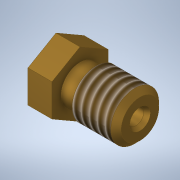
# Autodesk Inventor part: MINI-nozzle-0.4
Saved by Autodesk Inventor 2021 (Build 250183000, 183)
## iProperties
Company: Prusa Development a.s.
Created: 2019-02-18
Material: Všeobecné
Document SubType Name: Modeling
Density: 1 g/cm^3
Appearance: Mosaz – satén
Project: ORIGINAL PRUSA MINI
Authority: Ing. Robert Turinský
Author: Ing. Robert Turinský
Title: MINI-nozzle-0.4
Revision Number: R4
Autodesk Inventor part; units mm, degrees
ref_plane "YZ Plane" through (0, 0, 0) normal (1, 0, 0) x (0, 1, 0)
ref_plane "XZ Plane" through (0, 0, 0) normal (0, 1, 0) x (-1, 0, 0)
sketch "Náčrt1" plane through (0, 0, 0) normal (0, 0, 1) x (1, 0, 0)
  line L0 (0, -3.6) -> (0, 0.6) projected
  line L1 (-15, 0) -> (2.5, 0) projected
  line L2 (-0.5196, -1) -> (-10.5144, -1)
  line L3 (0, -1.3) -> (0, -3)
  line L4 (0, -3) -> (-5.5, -3)
  line L5 (-5.5, -3) -> (-6.1348, -1.9004)
  line L6 (-6.1348, -1.9004) -> (-10.5, -1.9004)
  line L7 (-10.5, -1.9004) -> (-12.5, -0.5)
  line L8 (-12.5, -0.5) -> (-12.5, -0.2)
  line L9 (-12.5, -0.2) -> (-11.9, -0.2)
  line L10 (-11.9, -0.2) -> (-10.5144, -1)
  line L11 (-0.5196, -1) -> (0, -1.3)
  line L12 (-5.8464, -2.4) -> (-7.5, -2.4)
  line L13 (-7.5, -2.4) -> (-7.5, -1.9004)
  point P0 (0, 0)
  dimension "d0" = 6
  dimension "d1" = 0.4
  dimension "d3" = 1
  dimension "d4" = 12.5
  dimension "d5" = 10.5
  dimension "d6" = 2
  dimension "d7" = 30
  dimension "d9" = 5.5
  dimension "d10" = 120
  dimension "d36" = 0.6
  dimension "d37" = 35
  dimension "d38" = 2.6
  dimension "d39" = 30
  dimension "d40" = 4.8
  dimension "d41" = 5
  constraints: 25 end point, 3 horizontal, 3 point on line, 2 perpendicular, 1 collinear, 1 parallel, 1 vertical
  measures "d0" diameter of L4 L1
  measures "d1" diameter of L9 L1
  measures "d3" diameter of L7.end L1
  measures "d4" distance between parallel lines of L0 L8
  measures "d5" distance from line of L0 L6.end
  measures "d6" diameter of L2 L1
  measures "d7" angle of L1 L10
  measures "d9" distance of L3.end L4.end
  measures "d10" angle of L4 L5
  measures "d36" distance of L8.end L9.end
  measures "d37" angle of L1 L7
  measures "d38" diameter of L3.start L1
  measures "d39" angle of L1 L11
  measures "d40" diameter of L12 L1
  measures "d41" distance between parallel lines of L13 L8
revolve "Rotace1" add sketch "Náčrt1" angle 360 about axis through (-10, 0, 0) along (1, 0, 0) contours L4 L5 L6 L7 L8 L9 L10 L2 L11 L0
ref_plane "Pracovní rovina1" through (-7.5, 0, 0) normal (1, 0, 0) x (0, 0, -1)
sketch "Náčrt2" plane through (-7.5, 0, 0) normal (1, 0, 0) x (0, 0, -1)
  line L0 (0, 4.0415) -> (3.5, 2.0207)
  line L1 (3.5, 2.0207) -> (3.5, -2.0207)
  line L2 (3.5, -2.0207) -> (0, -4.0415)
  line L3 (0, -4.0415) -> (-3.5, -2.0207)
  line L4 (-3.5, -2.0207) -> (-3.5, 2.0207)
  line L5 (-3.5, 2.0207) -> (0, 4.0415)
  circle A0 centre (0, 0) radius 1.9004 projected
  circle A1 centre (0, 0) radius 1.9004 projected
  dimension "d13" = 7
  constraints: 12 end point, 1 coincident, 1 vertical, 13 other
  measures "d13" distance between parallel lines of L1 L4
extrude "Vysunutí1" add sketch "Náčrt2" against normal blind 3
chamfer "Zkosení1" distance 0.65 angle 45 1 edges at (0, 3, 0)
thread "Závit1" size "M6x1" class "6g" standard "ANSI Metric M Profile" full length
fillet "Zaoblení1" radius 0.25 1 edges at (-10.5, 1.9004, 0)
sketch "Náčrt3" plane through (0, 0, 0) normal (0, 1, 0) x (-1, 0, 0)
  line L0 (7.5, 1.9004) -> (7.5, -1.9004) projected
  line L1 (7.5, 0) -> (7.5, -3.5) projected
  line L2 (7.5, 3.5) -> (7.5, 0) projected
  line L3 (7.5, 0) -> (7.5, 3.5) projected
  line L4 (7.5, -3.5) -> (7.5, 0) projected
  line L5 (10.5, 0) -> (10.5, -3.5) projected
  line L6 (10.5, -3.5) -> (10.5, 0) projected
  line L7 (10.5, 0) -> (10.5, 3.5) projected
  line L8 (10.5, 3.5) -> (10.5, 0) projected
  line L9 (10.5, -2.0306) -> (10.5, 2.0306) projected
  line L10 (7.5, 3.5) -> (10.5, 3.5) projected
  line L11 (7.5, 3.5) -> (10.5, 3.5) projected
  line L12 (12.6, 0) -> (-2.1, 0) projected
  line L13 (7.5, 3.625) -> (7.5, 4.5)
  line L14 (7.5, 4.5) -> (8.0052, 4.5)
  line L15 (8.0052, 4.5) -> (7.5, 3.625)
  line L16 (9, 3.5) -> (9, 2.759)
  line L17 (10.5, 3.625) -> (10.5, 4.5)
  line L18 (10.5, 4.5) -> (9.9948, 4.5)
  line L19 (9.9948, 4.5) -> (10.5, 3.625)
  point P0 (0, 0)
  dimension "d22" = 30
  dimension "d23" = 7.25
  dimension "d24" = 9
  constraints: 14 end point, 3 symmetric about line, 2 vertical, 1 collinear, 1 midpoint, 1 perpendicular
  measures "d22" angle of L13 L15
  measures "d23" diameter of L13.start L12
  measures "d24" diameter of L14 L12
revolve "Rotace2" [suppressed]
sketch "Náčrt4" plane through (0, 0, 0) normal (0, 1, 0) x (-1, 0, 0)
  line L0 (7.5, 3.5) -> (10.5, 3.5) projected
  line L1 (9, 3.5) -> (9, 2.8)
  line L2 (9, 2.8) -> (8.8264, 2.8)
  line L3 (8.8264, 2.8) -> (8.5, 3.5)
  line L4 (9, 3.5) -> (8.5, 3.5)
  point P0 (0, 0)
  point P1 (7.7404, 3.5)
  point P2 (10.2596, 3.5)
  dimension "d26" = 25
  dimension "d27" = 1
  dimension "d28" = 0.7
  constraints: 8 end point, 1 collinear, 1 midpoint, 1 perpendicular, 1 point on line, 1 vertical
  measures "d26" angle of L1 L3
  measures "d27" diameter of L3.end L1
  measures "d28" distance between parallel lines of L0 L2
revolve "Rotace3" [suppressed]
pattern_circular "Kruhové pole1" [suppressed]
revolve "Rotace4" add sketch "Náčrt1" angle 360 about axis through (-10, 0, 0) along (1, 0, 0) contours L12 L13 L6 L5
